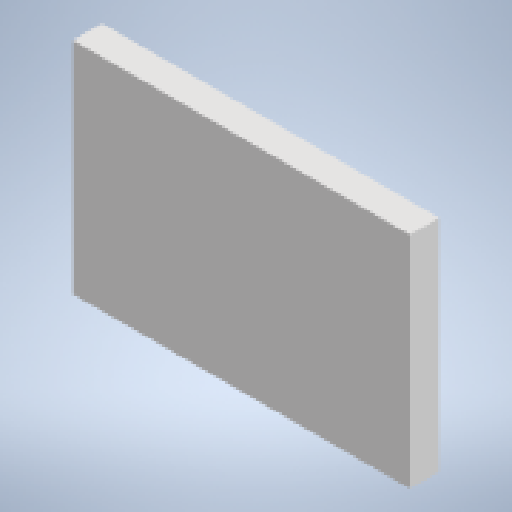
# Autodesk Inventor part: Light Pipe Translucent
Saved by Autodesk Inventor 2024 (Build 280153000, 153)
## iProperties
Created: 2024-06-30
Part Number: Light Pipe Translucent
Material: PET Plastic
Document SubType Name: Modeling
Designer: adam
Density: 1.541 g/cm^3
Appearance: Clear
Author: adam
Autodesk Inventor part; units mm, degrees
ref_plane "YZ Plane" through (0, 0, 0) normal (1, 0, 0) x (0, 1, 0)
ref_plane "XZ Plane" through (0, 0, 0) normal (0, 1, 0) x (-1, 0, 0)
ref_plane "XY Plane" through (0, 0, 0) normal (0, 0, 1) x (1, 0, 0)
sketch "Sketch1" plane through (0, 0, 0) normal (0, 0, 1) x (1, 0, 0)
  line L0 (-3, -1.125) -> (3, -1.125) construction
  line L1 (-3, -2) -> (3, -2) construction
  line L2 (-2.875, 1.875) -> (-2.875, -1.875)
  line L3 (-2.875, -1.875) -> (2.875, -1.875)
  line L4 (2.875, -1.875) -> (2.875, 1.875)
  line L5 (2.875, 1.875) -> (-2.875, 1.875)
  line L6 (-2.875, 1.875) -> (-2.875, 2) construction
  line L7 (-2.875, 1.875) -> (-3, 1.875) construction
  line L8 (-2.875, -1.875) -> (-2.875, -2) construction
  line L9 (3, -2) -> (3, -1.125) projected
  line L10 (-3, -1.125) -> (-3, -2) projected
  point P0 (0, 0)
  constraints: 14 end point, 5 perpendicular, 2 horizontal, 1 point on line
extrude "Extrusion1" add sketch "Sketch1" along normal blind 0.5
sketch "Sketch2" plane through (0, 0, 0) normal (0, 0, -1) x (-1, 0, 0)
  line L0 (2.875, 1.875) -> (2.875, -1.875) projected
  line L1 (-2.875, 1) -> (2.875, 1)
  line L2 (2.875, 1) -> (2.875, -1)
  line L3 (2.875, -1) -> (-2.875, -1)
  line L4 (-2.875, -1) -> (-2.875, 1)
  line L5 (-2.875, 1) -> (2.875, -1) construction
  line L6 (2.875, 1) -> (-2.875, -1) construction
  point P0 (0, 0)
  dimension "d2" = 2
  constraints: 12 end point, 2 midpoint, 2 parallel, 1 horizontal, 1 perpendicular, 1 point on line
  measures "d2" distance of L1.end L2.end
extrude "Extrusion2" add sketch "Sketch2" along normal blind 7
body "Solid1"
